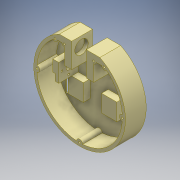
# Autodesk Inventor part: Cuerpo
Saved by Autodesk Inventor 2016 (Build 200138000, 138)
## iProperties
Created: 2019-03-15
Part Number: Cuerpo
Material: Nilón 6/6
Document SubType Name: Modeling
Designer: FIMCP
Mass: 170.58 g
Surface Area: 720.564 cm^2
Volume: 150.956 cm^3
Density: 1.13 g/cm^3
Appearance: Nilón 6
Author: FIMCP
Autodesk Inventor part; units mm, degrees
ref_plane "YZ Plane" through (0, 0, 0) normal (1, 0, 0) x (0, 1, 0)
ref_plane "XZ Plane" through (0, 0, 0) normal (0, 1, 0) x (-1, 0, 0)
ref_plane "XY Plane" through (0, 0, 0) normal (0, 0, 1) x (1, 0, 0)
sketch "Boceto1" plane through (0, 0, 0) normal (0, 1, 0) x (-1, 0, 0)
  arc A0 (-18, 72.808) -> (20, 72.2842) centre (0, 0) ccw
  line L0 (-18, 72.808) -> (-18, 72.2842)
  line L1 (-11, 25) -> (13, 25)
  line L2 (55, 8) -> (40, 8)
  line L3 (40, 8) -> (40, -42)
  line L4 (40, -42) -> (55, -42)
  line L5 (55, -42) -> (55, 8)
  line L6 (-40, 8) -> (-55, 8)
  line L7 (-55, 8) -> (-55, -42)
  line L8 (-55, -42) -> (-40, -42)
  line L9 (-40, -42) -> (-40, 8)
  line L10 (20, 72.2842) -> (13, 72.2842)
  line L11 (13, 72.2842) -> (13, 25)
  line L12 (-18, 72.808) -> (-11, 72.808)
  line L13 (-11, 72.808) -> (-11, 25)
  line L14 (-18, 72.2842) -> (-18, 72.808)
  dimension "d0" = 150
  dimension "d2" = 18
  dimension "d3" = 25
  dimension "d4" = 15
  dimension "d5" = 50
  dimension "d6" = 15
  dimension "d7" = 50
  dimension "d8" = 40
  dimension "d9" = 40
  dimension "d63" = 8
  dimension "d64" = 8
  constraints: 30 end point, 5 parallel, 4 horizontal, 4 perpendicular, 2 point on circle, 1 centre point, 1 coincident, 1 point on line
  measures "d0" diameter of A0
  measures "d2" distance from line of L0 point (0, 0)
  measures "d3" distance from line of L1 point (0, 0)
  measures "d4" distance of L4.end L3.end
  measures "d5" distance of L3.end L2.end
  measures "d6" distance of L8.end L7.end
  measures "d7" distance of L7.end L6.end
  measures "d8" distance from line of L9 point (0, 0)
  measures "d9" distance from line of L3 point (0, 0)
  measures "d63" distance from line of point (0, 0) L2
  measures "d64" distance from line of point (0, 0) L6
extrude "Extrusión1" add sketch "Boceto1" along normal blind 2
sketch "Boceto2" plane through (0, 0, 0) normal (0, 1, 0) x (-1, 0, 0)
  arc A0 (-18, 72.808) -> (20, 72.2842) centre (0, 0) ccw
  line L0 (-18, 72.808) -> (-18, 72.2842)
  line L1 (20, 72.2842) -> (13, 72.2842)
  line L2 (-18, 72.808) -> (-11, 72.808)
  line L3 (-11, 72.808) -> (-11, 72.2842)
  line L4 (-18, 72.2842) -> (-18, 72.808)
  line L5 (20, 72.2842) -> (13, 72.2842) projected
  line L6 (13, 72.2842) -> (20, 72.2842)
  line L7 (64.5832, 27.0002) -> (13, 27.0002)
  line L8 (13, 27.0002) -> (13, 72.2842)
  line L9 (-11, 72.2842) -> (-20, 72.2842)
  line L10 (-64.5832, 27.0002) -> (-11, 27.0002)
  line L11 (-11, 27.0002) -> (-11, 72.2842)
  arc A1 (69.8214, 4.9968) -> (69.8214, -4.9968) centre (70, 0) ccw
  arc A2 (-69.8214, -4.9968) -> (-69.8214, 4.9968) centre (-70, 0) ccw
  arc A3 (4.9968, -69.8214) -> (-4.9968, -69.8214) centre (0, -70) ccw
  arc A4 (4.9968, -69.8214) -> (69.8214, -4.9968) centre (0, 0) ccw
  arc A5 (69.8214, 4.9968) -> (64.5832, 27.0002) centre (0, 0) ccw
  arc A6 (-64.5832, 27.0002) -> (-69.8214, 4.9968) centre (0, 0) ccw
  arc A7 (-69.8214, -4.9968) -> (-4.9968, -69.8214) centre (0, 0) ccw
  dimension "d14" = 150
  dimension "d45" = 10
  dimension "d46" = 10
  dimension "d47" = 10
  constraints: 22 end point, 18 point on circle, 8 centre point, 4 horizontal, 3 parallel, 2 coincident, 2 point on line, 1 perpendicular
  measures "d14" diameter of A0
  measures "d45" diameter of A1
  measures "d46" diameter of A2
  measures "d47" diameter of A3
extrude "Extrusión2" add sketch "Boceto2" against normal blind 32 contours L9 L11 L10 A6 A2 A7 A3 A4 A1 A5 L7 L8 L1 A0
sketch "Boceto3" plane through (0, 0, 0) normal (0, 1, 0) x (-1, 0, 0)
  line L0 (-40, 8) -> (-40, -42) projected
  line L1 (-40, -3) -> (-15, -3)
  line L2 (-15, -3) -> (-15, -31)
  line L3 (-15, -31) -> (-40, -31)
  line L4 (-40, -31) -> (-40, -3)
  line L5 (39.9026, -3) -> (14.9026, -3)
  line L6 (14.9026, -3) -> (14.9026, -31)
  line L7 (14.9026, -31) -> (39.9026, -31)
  line L8 (39.9026, -31) -> (39.9026, -3)
  line L9 (-40, 8) -> (-55, 8) projected
  line L10 (55, 8) -> (40, 8) projected
  point P0 (0, 0)
  dimension "d27" = 25
  dimension "d28" = 28
  dimension "d30" = 25
  dimension "d31" = 28
  dimension "d65" = 11
  dimension "d66" = 11
  constraints: 16 end point, 4 parallel, 2 horizontal, 2 perpendicular, 1 point on line
  measures "d27" distance of L2.end L3.end
  measures "d28" distance of L1.end L2.end
  measures "d30" distance of L7.end L6.end
  measures "d31" distance of L6.end L5.end
  measures "d65" distance between parallel lines of L9 L1
  measures "d66" distance between parallel lines of L10 L5
extrude "Extrusión3" add sketch "Boceto3" against normal blind 11
sketch "Boceto4" plane through (0, 0, 0) normal (0, 1, 0) x (-1, 0, 0)
  line L0 (34, 26.7953) -> (43.9649, 26.7953)
  line L1 (43.9649, 26.7953) -> (43.9649, 8)
  line L2 (40, -2.9415) -> (34, -2.9415)
  line L3 (34, -2.9415) -> (34, 26.7953)
  line L4 (13, 27.0002) -> (13, 72.2842) projected
  line L5 (55, 8) -> (40, 8) projected
  line L6 (40, 8) -> (40, -42) projected
  line L7 (43.9649, 8) -> (40, 8)
  line L8 (40, 8) -> (40, -2.9415)
  line L9 (43.9649, 5.0585) -> (44, 5.0585)
  point P0 (0, 0)
  dimension "d37" = 21
  constraints: 14 end point, 3 parallel, 3 point on line, 2 horizontal, 2 perpendicular
  measures "d37" distance between parallel lines of L4 L3
extrude "Extrusión4" add sketch "Boceto4" against normal blind 32
sketch "Boceto5" plane through (0, 0, 0) normal (1, 0, 0) x (0, 1, 0)
  circle A0 centre (-16, 51.2842) radius 11
  line L0 (0, 72.2842) -> (-32, 72.2842) projected
  line L1 (2, -75) -> (2, 72.808) projected
  point P0 (0, 0)
  point P1 (2, 72.2842)
  dimension "d40" = 22
  dimension "d41" = 21
  dimension "d42" = 18
  constraints: 1 centre point
  measures "d40" diameter of A0
  measures "d41" distance from line of L0 A0.centre
  measures "d42" distance from line of L1 A0.centre
extrude "Extrusión5" cut sketch "Boceto5" along normal mid plane 38
sketch "Boceto6" plane through (0, 0, 0) normal (0, 1, 0) x (-1, 0, 0)
  arc A0 (69.8214, 4.9968) -> (69.8214, -4.9968) centre (70, 0) ccw projected
  circle A1 centre (70, 0) radius 1.5
  circle A2 centre (0, -70) radius 1.5
  circle A3 centre (-70, 0) radius 1.5
  line L0 (64.5832, 27.0002) -> (13, 27.0002) projected
  line L1 (-11, 27.0002) -> (-64.5832, 27.0002) projected
  point P0 (0, 0)
  dimension "d48" = 3
  dimension "d49" = 3
  dimension "d50" = 3
  constraints: 3 centre point, 1 coincident
  measures "d48" diameter of A1
  measures "d49" diameter of A2
  measures "d50" diameter of A3
extrude "Extrusión6" cut sketch "Boceto6" against normal blind 33
sketch "Boceto8" plane through (0, 0, 0) normal (0, 1, 0) x (-1, 0, 0)
  line L0 (59.5508, 67.2842) -> (-59.748, 67.2842)
  line L1 (-59.748, 67.2842) -> (-59.748, 82.2842)
  line L2 (-59.748, 82.2842) -> (59.5508, 82.2842)
  line L3 (59.5508, 82.2842) -> (59.5508, 67.2842)
  line L4 (13, 72.2842) -> (20, 72.2842) projected
  point P0 (0, 0)
  dimension "d67" = 15
  dimension "d71" = 5
  constraints: 8 end point, 2 parallel, 1 horizontal, 1 perpendicular
  measures "d67" distance of L0.end L1.end
  measures "d71" distance between parallel lines of L4 L0
extrude "Extrusión8" cut sketch "Boceto8" along normal mid plane 70
sketch "Boceto9" plane through (0, 0, 0) normal (0, 1, 0) x (-1, 0, 0)
  line L0 (-64.5832, 27.0002) -> (-11, 27.0002) projected
  line L1 (-23, 27.0002) -> (-64.5832, 27.0002)
  line L2 (-40.2309, 57.2842) -> (-23, 57.2842)
  line L3 (-23, 57.2842) -> (-23, 27.0002)
  line L4 (-11, 67.2842) -> (-11, 27.0002) projected
  line L5 (-33.1337, 67.2842) -> (-11, 67.2842) projected
  line L6 (25, 27.0002) -> (64.5832, 27.0002)
  line L7 (40.2309, 57.2842) -> (25, 57.2842)
  line L8 (25, 57.2842) -> (25, 27.0002)
  line L9 (13, 27.0002) -> (13, 67.2842) projected
  line L10 (13, 67.2842) -> (33.1337, 67.2842) projected
  arc A0 (-40.2309, 57.2842) -> (-64.5832, 27.0002) centre (0, 0) ccw
  arc A1 (64.5832, 27.0002) -> (40.2309, 57.2842) centre (0, 0) ccw
  dimension "d73" = 12
  dimension "d76" = 10
  dimension "d77" = 12
  dimension "d78" = 10
  constraints: 12 end point, 4 point on circle, 2 centre point, 2 horizontal, 2 parallel, 1 coincident, 1 point on line
  measures "d73" distance between parallel lines of L4 L3
  measures "d76" distance between parallel lines of L5 L2
  measures "d77" distance between parallel lines of L8 L9
  measures "d78" distance between parallel lines of L10 L7
extrude "Extrusión9" cut sketch "Boceto9" against normal blind 32
sketch "Boceto10" plane through (0, 0, 0) normal (0, 1, 0) x (-1, 0, 0)
  line L0 (-23, 57.2842) -> (-40.2309, 57.2842) projected
  circle A0 centre (-40.2309, 57.2842) radius 4
  arc A1 (69.8214, 4.9968) -> (40.2309, 57.2842) centre (0, 0) ccw projected
  circle A2 centre (40.2309, 57.2842) radius 4
  line L1 (25, 57.2842) -> (25, 27.0002) projected
  circle A3 centre (25, 57.2842) radius 4
  line L2 (-23, 27.0002) -> (-23, 57.2842) projected
  circle A4 centre (-23, 57.2842) radius 4
  line L3 (-11, 67.2842) -> (-11, 27.0002) projected
  dimension "d81" = 8
  dimension "d82" = 8
  dimension "d83" = 8
  dimension "d84" = 8
  constraints: 4 centre point, 1 coincident, 1 other
  measures "d81" diameter of A0
  measures "d82" diameter of A2
  measures "d83" diameter of A3
  measures "d84" diameter of A4
extrude "Extrusión10" add sketch "Boceto10" against normal blind 32
sketch "Boceto11" plane through (0, 0, 0) normal (0, 1, 0) x (-1, 0, 0)
  line L0 (-27, 57.2842) -> (-36.2309, 57.2842) projected
  arc A0 (-43.4373, 54.8927) -> (-36.2309, 57.2842) centre (-40.2309, 57.2842) ccw projected
  arc A1 (-27, 57.2842) -> (-23, 53.2842) centre (-23, 57.2842) ccw projected
  circle A2 centre (-23, 57.2842) radius 1.5
  arc A3 (25, 53.2842) -> (29, 57.2842) centre (25, 57.2842) ccw projected
  circle A4 centre (25, 57.2842) radius 1.5
  arc A5 (36.2309, 57.2842) -> (43.4373, 54.8927) centre (40.2309, 57.2842) ccw projected
  circle A6 centre (40.2309, 57.2842) radius 1.5
  circle A7 centre (-40.2309, 57.2842) radius 1.5
  point P0 (0, 0)
  dimension "d89" = 3
  dimension "d90" = 3
  dimension "d91" = 3
  dimension "d92" = 3
  constraints: 4 centre point, 4 coincident
  measures "d89" diameter of A2
  measures "d90" diameter of A4
  measures "d91" diameter of A6
  measures "d92" diameter of A7
extrude "Extrusión11" cut sketch "Boceto11" against normal blind 32
sketch "Boceto12" plane through (0, 0, 0) normal (1, 0, 0) x (0, 1, 0)
  circle A0 centre (-16, 12.0585) radius 4
  line L0 (0, 54.8927) -> (0, 4.9968) projected
  line L1 (0, -2.9415) -> (-32, -2.9415) projected
  circle A1 centre (-5, 12.0585) radius 1.5
  line L2 (-32, 67.2842) -> (-32, -75) projected
  circle A2 centre (-27, 12.0585) radius 1.5
  circle A3 centre (-16, 2.0585) radius 1.5
  circle A4 centre (-16, 20.5585) radius 1.5
  point P0 (0, 0)
  dimension "d95" = 8
  dimension "d96" = 16
  dimension "d97" = 15
  dimension "d98" = 3
  dimension "d99" = 5
  dimension "d102" = 3
  dimension "d103" = 5
  dimension "d104" = 3
  dimension "d105" = 5
  dimension "d106" = 3
  dimension "d107" = 16
  dimension "d108" = 16
  dimension "d109" = 15
  dimension "d110" = 23.5
  constraints: 5 centre point
  measures "d95" diameter of A0
  measures "d96" distance from line of A0.centre L0
  measures "d97" distance from line of L1 A0.centre
  measures "d98" diameter of A1
  measures "d99" distance from line of L0 A1.centre
  measures "d102" diameter of A2
  measures "d103" distance from line of L2 A2.centre
  measures "d104" diameter of A3
  measures "d105" distance from line of L1 A3.centre
  measures "d106" diameter of A4
  measures "d107" distance from line of L0 A3.centre
  measures "d108" distance from line of L0 A4.centre
  measures "d109" distance from line of L1 A2.centre
  measures "d110" distance from line of L1 A4.centre
extrude "Extrusión12" cut sketch "Boceto12" against normal blind 50
sketch "Boceto13" plane through (0, 0, 0) normal (0, 1, 0) x (-1, 0, 0)
  line L0 (-11, 67.2842) -> (-11, 27.0002) projected
  line L1 (-19, 62.2842) -> (-19, 40.2842) projected
  line L2 (-11, 62.2842) -> (-19, 62.2842)
  line L3 (-19, 62.2842) -> (-19, 40.2842)
  line L4 (-19, 40.2842) -> (-11, 40.2842)
  line L5 (-11, 40.2842) -> (-11, 62.2842)
  point P0 (0, 0)
  constraints: 8 end point, 2 parallel, 1 horizontal, 1 perpendicular, 1 point on line
extrude "Extrusión13" cut sketch "Boceto13" along normal mid plane 32
sketch "Boceto14" plane through (0, 0, 0) normal (1, 0, 0) x (0, 1, 0)
  circle A0 centre (-2, 55.2842) radius 1.5
  line L0 (2, -75) -> (2, 67.2842) projected
  line L1 (2, 67.2842) -> (-32, 67.2842) projected
  circle A1 centre (-2, 47.2842) radius 1.5
  point P0 (0, 0)
  dimension "d118" = 3
  dimension "d119" = 4
  dimension "d120" = 12
  dimension "d121" = 3
  dimension "d122" = 4
  dimension "d123" = 20
  constraints: 2 centre point
  measures "d118" diameter of A0
  measures "d119" distance from line of L0 A0.centre
  measures "d120" distance from line of L1 A0.centre
  measures "d121" diameter of A1
  measures "d122" distance from line of A1.centre L0
  measures "d123" distance from line of L1 A1.centre
extrude "Extrusión14" cut sketch "Boceto14" along normal blind 29
